Autodesk Fusion 360 part; units mm, degrees
note: some values were not read from the file. Chosen so that the rebuilt part matches the saved one: which face or edge a step refers to; which pieces of a blend or face edit are solid. Set by a fixed rule: which sketch regions a step uses.
(part 4 of 5)
  line L270 (74.1186, 72.7044) -> (69.1688, 67.7546)
  line L271 (49.0163, 92.8569) -> (45.9408, 89.7814)
  line L272 (61.3906, 64.2191) -> (67.0475, 69.8759)
  line L273 (69.8759, 67.0475) -> (64.2191, 61.3906)
  line L274 (70.9366, 70.9366) -> (49.0163, 92.8569)
  line L275 (56.4409, 62.0978) -> (59.9764, 65.6333)
  line L276 (70.9366, 70.9366) -> (49.0163, 92.8569)
  line L277 (69.8759, 67.0475) -> (64.2191, 61.3906)
  arc A224 (33.8135, 84.7252) -> (33.8135, 77.6541) centre (37.349, 81.1896) ccw
  arc A225 (37.0951, 88.0068) -> (35.2806, 96.2368) centre (33.5596, 91.5424) ccw
  line L278 (38.7632, 55.7338) -> (34.8741, 51.8447)
  arc A226 (37.0951, 88.0068) -> (35.2806, 96.2368) centre (33.5596, 91.5424) ccw
  arc A227 (40.8846, 84.7252) -> (40.8846, 77.6541) centre (44.4201, 81.1896) ccw
  arc A228 (40.8846, 84.7252) -> (40.8846, 77.6541) centre (44.4201, 81.1896) ccw
  line L279 (38.7632, 55.7338) -> (34.8741, 51.8447)
  line L280 (33.8135, 84.7252) -> (37.0951, 88.0068)
  line L281 (49.7234, 68.8153) -> (40.8846, 77.6541)
  line L282 (33.8135, 84.7252) -> (37.0951, 88.0068)
  arc A229 (33.8135, 84.7252) -> (33.8135, 77.6541) centre (37.349, 81.1896) ccw
  arc A230 (77.6541, 40.8846) -> (84.7252, 40.8846) centre (81.1896, 44.4201) ccw
  line L283 (49.0163, 92.8569) -> (45.9408, 89.7814)
  arc A231 (99.7259, 40.1371) -> (86.6476, 42.807) centre (92.3045, 37.1501) ccw
  line L284 (67.0475, 69.8759) -> (69.8759, 67.0475)
  arc A232 (24.049, -81.3368) -> (30.5907, -80.8769) centre (27.0551, -77.3414) ccw
  arc A233 (77.6541, 40.8846) -> (84.7252, 40.8846) centre (81.1896, 44.4201) ccw
  line L285 (88.4889, 37.5772) -> (86.1394, 35.2277)
  arc A234 (96.2368, 35.2806) -> (88.0068, 37.0951) centre (91.5424, 33.5596) ccw
  line L286 (61.3906, 64.2191) -> (67.0475, 69.8759)
  line L287 (74.1186, 72.7044) -> (69.1688, 67.7546)
  arc A235 (45.9408, 89.7814) -> (44.4738, 97.869) centre (42.4052, 93.3169) ccw
  line L288 (72.7044, 74.1186) -> (74.1186, 72.7044)
  circle A236 centre (64.2191, 64.2191) radius 1
  line L289 (92.8569, 49.0163) -> (70.9366, 70.9366)
  line L290 (49.7234, 68.8153) -> (68.8153, 49.7234)
  line L291 (65.6333, 59.9764) -> (62.0978, 56.4409)
  circle A237 centre (27.9799, -51.6679) radius 1.75
  line L292 (-80.8769, 30.5907) -> (-81.1896, 30.278)
  line L293 (-51.8447, -34.8741) -> (-34.8741, -51.8447)
  line L294 (-86.1394, 35.2277) -> (-84.7252, 33.8135)
  line L295 (-56.4409, -62.0978) -> (-40.8846, -77.6541)
  line L296 (-37.7026, -56.7945) -> (-56.7945, -37.7026)
  line L297 (-37.7026, -56.7945) -> (-56.7945, -37.7026)
  line L298 (-39.8239, -11.5396) -> (-57.5016, -29.2173)
  line L299 (-11.5396, -39.8239) -> (-39.8239, -11.5396)
  line L300 (-68.8153, -49.7234) -> (-49.7234, -68.8153)
  line L301 (-39.8239, -11.5396) -> (-57.5016, -29.2173)
  line L302 (-80.8769, 30.5907) -> (-81.1896, 30.278)
  line L303 (-30.5907, -80.8769) -> (-77.6541, -33.8135)
  arc A238 (-30.5907, -80.8769) -> (-24.049, -81.3368) centre (-27.0551, -77.3414) ccw
  line L304 (-29.2173, -57.5016) -> (-11.5396, -39.8239)
  line L305 (-11.5396, -39.8239) -> (-39.8239, -11.5396)
  line L306 (-57.5016, -29.2173) -> (-29.2173, -57.5016)
  arc A239 (-44.4738, -97.869) -> (-37.8014, -100.6345) centre (0, 0) ccw
  line L307 (-56.4409, -62.0978) -> (-40.8846, -77.6541)
  line L308 (-56.4409, -62.0978) -> (-62.0978, -56.4409)
  arc A240 (-44.4738, -97.869) -> (-37.8014, -100.6345) centre (0, 0) ccw
  line L309 (-51.8447, -34.8741) -> (-34.8741, -51.8447)
  line L310 (-49.7234, -68.8153) -> (-37.7026, -56.7945)
  line L311 (-34.8741, -51.8447) -> (-38.7632, -55.7338)
  line L312 (-30.5907, -80.8769) -> (-77.6541, -33.8135)
  line L313 (-51.8447, -34.8741) -> (-34.8741, -51.8447)
  circle A241 centre (-41.0613, -17.3733) radius 1.75
  line L314 (-34.8741, -51.8447) -> (-38.7632, -55.7338)
  line L315 (-57.5016, -29.2173) -> (-29.2173, -57.5016)
  line L316 (-38.7632, -55.7338) -> (-55.7338, -38.7632)
  line L317 (-51.8447, -34.8741) -> (-34.8741, -51.8447)
  line L318 (-38.7632, -55.7338) -> (-55.7338, -38.7632)
  line L319 (-86.1394, 35.2277) -> (-84.7252, 33.8135)
  circle A242 centre (-41.0613, -17.3733) radius 1.75
  arc A243 (-42.807, -86.6476) -> (-40.1371, -99.7259) centre (-37.1501, -92.3045) ccw
  line L320 (-29.2173, -57.5016) -> (-11.5396, -39.8239)
  line L321 (-29.2173, -57.5016) -> (-11.5396, -39.8239)
  line L322 (-34.8741, -51.8447) -> (-38.7632, -55.7338)
  circle A244 centre (-41.0613, -17.3733) radius 1.75
  line L323 (-37.7026, -56.7945) -> (-56.7945, -37.7026)
  circle A245 centre (-17.3733, -41.0613) radius 1.75
  circle A246 centre (-41.0613, -17.3733) radius 1.75
  line L324 (-11.5396, -39.8239) -> (-39.8239, -11.5396)
  line L325 (-39.8239, -11.5396) -> (-57.5016, -29.2173)
  line L326 (-51.8447, -34.8741) -> (-34.8741, -51.8447)
  line L327 (-34.8741, -51.8447) -> (-38.7632, -55.7338)
  arc A247 (-44.4738, -97.869) -> (-37.8014, -100.6345) centre (0, 0) ccw
  line L328 (-38.7632, -55.7338) -> (-55.7338, -38.7632)
  line L329 (-34.8741, -51.8447) -> (-38.7632, -55.7338)
  line L330 (-11.5396, -39.8239) -> (-39.8239, -11.5396)
  circle A248 centre (-27.9799, -51.6679) radius 1.75
  line L331 (-56.4409, -62.0978) -> (-40.8846, -77.6541)
  line L332 (-88.4889, 37.5772) -> (-86.1394, 35.2277)
  line L333 (-86.1394, 35.2277) -> (-84.7252, 33.8135)
  line L334 (-39.8239, -11.5396) -> (-57.5016, -29.2173)
  line L335 (-38.7632, -55.7338) -> (-55.7338, -38.7632)
  line L336 (-34.8741, -51.8447) -> (-38.7632, -55.7338)
  line L337 (-41.5917, -85.4323) -> (-49.0163, -92.8569)
  line L338 (-83.0899, 32.1782) -> (-81.1896, 30.278)
  line L339 (-38.7632, -55.7338) -> (-55.7338, -38.7632)
  line L340 (-34.8741, -51.8447) -> (-38.7632, -55.7338)
  line L341 (-57.5016, -29.2173) -> (-29.2173, -57.5016)
  circle A249 centre (-27.9799, -51.6679) radius 1.75
  line L342 (-38.7632, -55.7338) -> (-55.7338, -38.7632)
  circle A250 centre (-41.0613, -17.3733) radius 1.75
  arc A251 (0, -78.3) -> (-31.5378, -98.1221) centre (0, -113.3) ccw
  line L343 (-68.8153, -49.7234) -> (-49.7234, -68.8153)
  line L344 (-70.9366, -70.9366) -> (-92.8569, -49.0163)
  line L345 (-65.6333, -59.9764) -> (-59.9764, -65.6333)
  line L346 (-37.5772, -88.4889) -> (-35.2277, -86.1394)
  arc A252 (0, -78.3) -> (-31.5378, -98.1221) centre (0, -113.3) ccw
  arc A253 (-31.8637, -89.1193) -> (-35.2447, -94.3842) centre (0, -113.3) ccw
  arc A254 (0, -73.3) -> (-24.049, -81.3368) centre (0, -113.3) ccw
  circle A255 centre (-17.3733, -41.0613) radius 1.75
  arc A256 (24.049, -81.3368) -> (0, -73.3) centre (0, -113.3) ccw
  line L347 (-56.4409, -62.0978) -> (-62.0978, -56.4409)
  line L348 (-68.8153, -49.7234) -> (-49.7234, -68.8153)
  line L349 (-56.4409, -62.0978) -> (-62.0978, -56.4409)
  arc A257 (0, -73.3) -> (-24.049, -81.3368) centre (0, -113.3) ccw
  line L350 (-41.5917, -85.4323) -> (-40.8846, -84.7252)
  line L351 (-32.3993, -86.1394) -> (-32.0426, -86.496)
  arc A258 (-31.8637, -89.1193) -> (-35.2447, -94.3842) centre (0, -113.3) ccw
  line L352 (-65.6333, -59.9764) -> (-59.9764, -65.6333)
  line L353 (-56.4409, -62.0978) -> (-62.0978, -56.4409)
  circle A259 centre (-17.3733, -41.0613) radius 1.75
  arc A260 (-31.8637, -89.1193) -> (-35.2447, -94.3842) centre (0, -113.3) ccw
  arc A261 (24.049, -81.3368) -> (0, -73.3) centre (0, -113.3) ccw
  arc A262 (0, -73.3) -> (-24.049, -81.3368) centre (0, -113.3) ccw
  line L354 (-37.5772, -88.4889) -> (-40.3326, -91.2443)
  line L355 (-68.8153, -49.7234) -> (-49.7234, -68.8153)
  line L356 (-65.6333, -59.9764) -> (-59.9764, -65.6333)
  line L357 (-56.4409, -62.0978) -> (-62.0978, -56.4409)
  line L358 (-65.6333, -59.9764) -> (-59.9764, -65.6333)
  line L359 (-70.9366, -70.9366) -> (-92.8569, -49.0163)
  line L360 (-70.9366, -70.9366) -> (-92.8569, -49.0163)
  arc A263 (24.049, -81.3368) -> (0, -73.3) centre (0, -113.3) ccw
  arc A264 (24.049, -81.3368) -> (0, -73.3) centre (0, -113.3) ccw
  circle A265 centre (-27.9799, -51.6679) radius 1.75
  arc A266 (-31.321, -97.5974) -> (-31.2855, -97.6087) centre (0, 0) ccw
  line L361 (-29.2173, -57.5016) -> (-11.5396, -39.8239)
  line L362 (-65.6333, -59.9764) -> (-59.9764, -65.6333)
  circle A267 centre (-17.3733, -41.0613) radius 1.75
  circle A268 centre (-27.9799, -51.6679) radius 1.75
  line L363 (-37.5772, -88.4889) -> (-40.3326, -91.2443)
  line L364 (-68.8153, -49.7234) -> (-49.7234, -68.8153)
  arc A269 (0, -73.3) -> (-24.049, -81.3368) centre (0, -113.3) ccw
  line L365 (-70.9366, -70.9366) -> (-92.8569, -49.0163)
  line L366 (-37.5772, -88.4889) -> (-40.3326, -91.2443)
  arc A270 (0, -73.3) -> (-24.049, -81.3368) centre (0, -113.3) ccw
  line L367 (-37.5772, -88.4889) -> (-40.3326, -91.2443)
  arc A271 (-30.5907, -80.8769) -> (-24.049, -81.3368) centre (-27.0551, -77.3414) ccw
  line L368 (-65.6333, -59.9764) -> (-59.9764, -65.6333)
  arc A272 (0, -73.3) -> (-24.049, -81.3368) centre (0, -113.3) ccw
  arc A273 (-40.8846, -84.7252) -> (-40.8846, -77.6541) centre (-44.4201, -81.1896) ccw
  line L369 (-68.8153, -49.7234) -> (-49.7234, -68.8153)
  line L370 (-65.6333, -59.9764) -> (-59.9764, -65.6333)
  line L371 (-41.5917, -85.4323) -> (-40.8846, -84.7252)
  line L372 (-34.8741, -51.8447) -> (-38.7632, -55.7338)
  arc A274 (-32.3993, -86.1394) -> (-35.2277, -86.1394) centre (-33.8135, -87.5536) ccw
  arc A275 (24.049, -81.3368) -> (0, -73.3) centre (0, -113.3) ccw
  arc A276 (-31.8637, -89.1193) -> (-35.2447, -94.3842) centre (0, -113.3) ccw
  arc A277 (24.049, -81.3368) -> (0, -73.3) centre (0, -113.3) ccw
  arc A278 (-37.7434, -95.2979) -> (-35.2447, -94.3842) centre (-37.007, -93.4384) ccw
  arc A279 (-37.9256, -100.5859) -> (-37.9262, -100.5876) centre (0, -113.3) ccw
  line L373 (-65.6333, -59.9764) -> (-59.9764, -65.6333)
  line L374 (-68.8153, -49.7234) -> (-49.7234, -68.8153)
  line L375 (-56.4409, -62.0978) -> (-62.0978, -56.4409)
  line L376 (-38.7632, -55.7338) -> (-55.7338, -38.7632)
  line L377 (-56.4409, -62.0978) -> (-62.0978, -56.4409)
  arc A280 (-40.3326, -91.2443) -> (-39.6929, -94.5025) centre (-38.9184, -92.6585) ccw
  arc A281 (-40.8846, -84.7252) -> (-40.8846, -77.6541) centre (-44.4201, -81.1896) ccw
  arc A282 (-37.9256, -100.5859) -> (-37.9262, -100.5876) centre (0, -113.3) ccw
  line L378 (-56.7945, -37.7026) -> (-68.8153, -49.7234)
  line L379 (-37.5772, -88.4889) -> (-35.2277, -86.1394)
  line L380 (-59.9764, -65.6333) -> (-56.4409, -62.0978)
  arc A283 (-40.3326, -91.2443) -> (-39.6929, -94.5025) centre (-38.9184, -92.6585) ccw
  arc A284 (-31.8637, -89.1193) -> (-32.0426, -86.496) centre (-33.4568, -87.9102) ccw
  arc A285 (-31.8637, -89.1193) -> (-32.0426, -86.496) centre (-33.4568, -87.9102) ccw
  arc A286 (-37.9256, -100.5859) -> (-37.9262, -100.5876) centre (0, -113.3) ccw
  arc A287 (-37.9256, -100.5859) -> (-37.9262, -100.5876) centre (0, -113.3) ccw
  line L381 (-56.7945, -37.7026) -> (-68.8153, -49.7234)
  arc A288 (-39.6929, -94.5025) -> (-37.7434, -95.2979) centre (0, 0) ccw
  arc A289 (-39.6929, -94.5025) -> (-37.7434, -95.2979) centre (0, 0) ccw
  line L382 (-59.9764, -65.6333) -> (-56.4409, -62.0978)
  arc A290 (-32.3993, -86.1394) -> (-35.2277, -86.1394) centre (-33.8135, -87.5536) ccw
  line L383 (-69.8759, -67.0475) -> (-67.0475, -69.8759)
  line L384 (-56.7945, -37.7026) -> (-68.8153, -49.7234)
  arc A291 (-37.7434, -95.2979) -> (-35.2447, -94.3842) centre (-37.007, -93.4384) ccw
  line L385 (-56.7945, -37.7026) -> (-68.8153, -49.7234)
  arc A292 (-32.3993, -86.1394) -> (-35.2277, -86.1394) centre (-33.8135, -87.5536) ccw
  line L386 (-56.7945, -37.7026) -> (-68.8153, -49.7234)
  line L387 (-56.7945, -37.7026) -> (-68.8153, -49.7234)
  line L388 (-59.9764, -65.6333) -> (-56.4409, -62.0978)
  line L389 (-49.0163, -92.8569) -> (-70.9366, -70.9366)
  line L390 (-68.8153, -49.7234) -> (-49.7234, -68.8153)
  line L391 (-59.9764, -65.6333) -> (-56.4409, -62.0978)
  line L392 (-49.0163, -92.8569) -> (-45.9408, -89.7814)
  arc A293 (-31.8637, -89.1193) -> (-32.0426, -86.496) centre (-33.4568, -87.9102) ccw
  line L393 (-41.5917, -85.4323) -> (-40.8846, -84.7252)
  line L394 (-59.9764, -65.6333) -> (-56.4409, -62.0978)
  line L395 (-49.0163, -92.8569) -> (-70.9366, -70.9366)
  arc A294 (-39.6929, -94.5025) -> (-37.7434, -95.2979) centre (0, 0) ccw
  line L396 (-56.7945, -37.7026) -> (-68.8153, -49.7234)
  line L397 (-64.2191, -61.3906) -> (-69.8759, -67.0475)
  line L398 (-59.9764, -65.6333) -> (-56.4409, -62.0978)
  arc A295 (-37.9256, -100.5859) -> (-37.9262, -100.5876) centre (0, -113.3) ccw
  arc A296 (-40.3326, -91.2443) -> (-39.6929, -94.5025) centre (-38.9184, -92.6585) ccw
  line L399 (-32.3993, -86.1394) -> (-32.0426, -86.496)
  line L400 (-49.0163, -92.8569) -> (-70.9366, -70.9366)
  arc A297 (-37.7434, -95.2979) -> (-35.2447, -94.3842) centre (-37.007, -93.4384) ccw
  line L401 (-41.5917, -85.4323) -> (-40.8846, -84.7252)
  arc A298 (-39.6929, -94.5025) -> (-37.7434, -95.2979) centre (0, 0) ccw
  arc A299 (-37.9256, -100.5859) -> (-37.9262, -100.5876) centre (0, -113.3) ccw
  line L402 (-59.9764, -65.6333) -> (-56.4409, -62.0978)
  line L403 (-37.5772, -88.4889) -> (-35.2277, -86.1394)
  arc A300 (-37.7434, -95.2979) -> (-35.2447, -94.3842) centre (-37.007, -93.4384) ccw
  arc A301 (-40.8846, -84.7252) -> (-40.8846, -77.6541) centre (-44.4201, -81.1896) ccw
  arc A302 (-40.3326, -91.2443) -> (-39.6929, -94.5025) centre (-38.9184, -92.6585) ccw
  arc A303 (-32.3993, -86.1394) -> (-35.2277, -86.1394) centre (-33.8135, -87.5536) ccw
  arc A304 (-31.8637, -89.1193) -> (-32.0426, -86.496) centre (-33.4568, -87.9102) ccw
  line L404 (-37.5772, -88.4889) -> (-35.2277, -86.1394)
  arc A305 (-31.321, -97.5974) -> (-31.2855, -97.6087) centre (0, 0) ccw
  line L405 (-56.7945, -37.7026) -> (-68.8153, -49.7234)
  line L406 (-49.0163, -92.8569) -> (-70.9366, -70.9366)
  line L407 (-32.3993, -86.1394) -> (-32.0426, -86.496)
  line L408 (-64.2191, -61.3906) -> (-69.8759, -67.0475)
  line L409 (-56.4409, -62.0978) -> (-62.0978, -56.4409)
  line L410 (-32.3993, -86.1394) -> (-32.0426, -86.496)
  arc A306 (-40.8846, -84.7252) -> (-40.8846, -77.6541) centre (-44.4201, -81.1896) ccw
  line L411 (-49.0163, -92.8569) -> (-42.807, -86.6476)
  circle A307 centre (-51.6679, -27.9799) radius 1.75
  arc A308 (-45.9408, -89.7814) -> (-44.4738, -97.869) centre (-42.4052, -93.3169) ccw
  arc A309 (-37.9256, -100.5859) -> (-37.9262, -100.5876) centre (0, -113.3) ccw
  arc A310 (-31.321, -97.5974) -> (-31.2855, -97.6087) centre (0, 0) ccw
  line L412 (-55.7338, -38.7632) -> (-51.8447, -34.8741)
  arc A311 (-37.9256, -100.5859) -> (-31.321, -97.5974) centre (-36.0432, -95.9538) ccw
  circle A312 centre (-51.6679, -27.9799) radius 1.75
  line L413 (-55.7338, -38.7632) -> (-51.8447, -34.8741)
  arc A313 (-31.321, -97.5974) -> (-31.2855, -97.6087) centre (0, 0) ccw
  line L414 (-64.2191, -61.3906) -> (-69.8759, -67.0475)
  line L415 (-92.8569, -49.0163) -> (-84.7252, -40.8846)
  line L416 (-69.8759, -67.0475) -> (-67.0475, -69.8759)
  line L417 (-92.8569, -49.0163) -> (-84.7252, -40.8846)
  line L418 (-64.2191, -61.3906) -> (-69.8759, -67.0475)
  line L419 (-92.8569, -49.0163) -> (-84.7252, -40.8846)
  arc A314 (-31.321, -97.5974) -> (-31.2855, -97.6087) centre (0, 0) ccw
  line L420 (-49.0163, -92.8569) -> (-45.9408, -89.7814)
  arc A315 (-96.2368, -35.2806) -> (-88.0068, -37.0951) centre (-91.5424, -33.5596) ccw
  line L421 (-69.8759, -67.0475) -> (-67.0475, -69.8759)
  arc A316 (-37.9256, -100.5859) -> (-37.9262, -100.5876) centre (0, -113.3) ccw
  line L422 (-55.7338, -38.7632) -> (-51.8447, -34.8741)
  line L423 (-92.8569, -49.0163) -> (-86.6476, -42.807)
  line L424 (-64.2191, -61.3906) -> (-69.8759, -67.0475)
  line L425 (-49.0163, -92.8569) -> (-45.9408, -89.7814)
  arc A317 (-45.9408, -89.7814) -> (-44.4738, -97.869) centre (-42.4052, -93.3169) ccw
  line L426 (-84.7252, -33.8135) -> (-88.0068, -37.0951)
  line L427 (-55.7338, -38.7632) -> (-51.8447, -34.8741)
  line L428 (-55.7338, -38.7632) -> (-51.8447, -34.8741)
  circle A318 centre (-64.2191, -64.2191) radius 1
  line L429 (-55.7338, -38.7632) -> (-51.8447, -34.8741)
  line L430 (-67.0475, -69.8759) -> (-61.3906, -64.2191)
  arc A319 (-37.9256, -100.5859) -> (-37.9262, -100.5876) centre (0, -113.3) ccw
  line L431 (-69.8759, -67.0475) -> (-67.0475, -69.8759)
  circle A320 centre (-51.6679, -27.9799) radius 1.75
  line L432 (-49.0163, -92.8569) -> (-45.9408, -89.7814)
  circle A321 centre (-51.6679, -27.9799) radius 1.75
  line L433 (-84.7252, -33.8135) -> (-88.0068, -37.0951)
  arc A322 (-31.321, -97.5974) -> (-31.2855, -97.6087) centre (0, 0) ccw
  arc A323 (-37.9256, -100.5859) -> (-31.321, -97.5974) centre (-36.0432, -95.9538) ccw
  arc A324 (-45.9408, -89.7814) -> (-44.4738, -97.869) centre (-42.4052, -93.3169) ccw
  line L434 (-92.8569, -49.0163) -> (-85.4323, -41.5917)
  circle A325 centre (-51.6679, -27.9799) radius 1.75
  line L435 (-69.8759, -67.0475) -> (-67.0475, -69.8759)
  arc A326 (-37.9256, -100.5859) -> (-37.9262, -100.5876) centre (0, -113.3) ccw
  line L436 (-69.8759, -67.0475) -> (-67.0475, -69.8759)
  line L437 (-59.9764, -65.6333) -> (-56.4409, -62.0978)
  line L438 (-84.7252, -33.8135) -> (-88.0068, -37.0951)
  line L439 (-69.8759, -67.0475) -> (-67.0475, -69.8759)
  line L440 (-55.7338, -38.7632) -> (-51.8447, -34.8741)
  line L441 (-69.8759, -67.0475) -> (-67.0475, -69.8759)
  line L442 (-64.2191, -61.3906) -> (-69.8759, -67.0475)
  arc A327 (-37.9256, -100.5859) -> (-37.9262, -100.5876) centre (0, -113.3) ccw
  circle A328 centre (-51.6679, -27.9799) radius 1.75
  circle A329 centre (-51.6679, -27.9799) radius 1.75
  arc A330 (-31.321, -97.5974) -> (-31.2855, -97.6087) centre (0, 0) ccw
  arc A331 (-37.9256, -100.5859) -> (-37.9262, -100.5876) centre (0, -113.3) ccw
  line L443 (-92.8569, -49.0163) -> (-85.4323, -41.5917)
  arc A332 (-45.9408, -89.7814) -> (-44.4738, -97.869) centre (-42.4052, -93.3169) ccw
  arc A333 (-37.9256, -100.5859) -> (-31.321, -97.5974) centre (-36.0432, -95.9538) ccw
  arc A334 (-31.321, -97.5974) -> (-31.2855, -97.6087) centre (0, 0) ccw
  line L444 (-92.8569, -49.0163) -> (-85.4323, -41.5917)
  arc A335 (-37.9256, -100.5859) -> (-31.321, -97.5974) centre (-36.0432, -95.9538) ccw
  arc A336 (-96.2368, -35.2806) -> (-88.0068, -37.0951) centre (-91.5424, -33.5596) ccw
  line L445 (-64.2191, -61.3906) -> (-69.8759, -67.0475)
  line L446 (-55.7338, -38.7632) -> (-51.8447, -34.8741)
  circle A337 centre (-51.6679, -27.9799) radius 1.75
  line L447 (-64.2191, -61.3906) -> (-69.8759, -67.0475)
  circle A338 centre (-64.2191, -64.2191) radius 1
  line L448 (-61.3906, -64.2191) -> (-64.2191, -61.3906)
  arc A339 (-96.2368, -35.2806) -> (-88.0068, -37.0951) centre (-91.5424, -33.5596) ccw
  line L449 (-61.3906, -64.2191) -> (-64.2191, -61.3906)
  circle A340 centre (-64.2191, -64.2191) radius 1
  line L450 (-92.8569, -49.0163) -> (-89.7814, -45.9408)
  line L451 (-61.3906, -64.2191) -> (-64.2191, -61.3906)
  line L452 (-69.1688, -67.7546) -> (-74.1186, -72.7044)
  arc A341 (-97.869, -44.4738) -> (-89.7814, -45.9408) centre (-93.3169, -42.4052) ccw
  line L453 (-61.3906, -64.2191) -> (-64.2191, -61.3906)
  line L454 (-62.0978, -56.4409) -> (-65.6333, -59.9764)
  line L455 (-69.1688, -67.7546) -> (-74.1186, -72.7044)
  line L456 (-67.0475, -69.8759) -> (-61.3906, -64.2191)
  line L457 (-62.0978, -56.4409) -> (-65.6333, -59.9764)
  line L458 (-72.7044, -74.1186) -> (-67.7546, -69.1688)
  line L459 (-62.0978, -56.4409) -> (-65.6333, -59.9764)
  circle A342 centre (-64.2191, -64.2191) radius 1
  line L460 (-72.7044, -74.1186) -> (-67.7546, -69.1688)
  line L461 (-69.1688, -67.7546) -> (-74.1186, -72.7044)
  line L462 (-67.0475, -69.8759) -> (-61.3906, -64.2191)
  line L463 (-62.0978, -56.4409) -> (-65.6333, -59.9764)
  line L464 (-72.7044, -74.1186) -> (-67.7546, -69.1688)
  line L465 (-68.8153, -49.7234) -> (-77.6541, -40.8846)
  line L466 (-62.0978, -56.4409) -> (-65.6333, -59.9764)
  arc A343 (-96.2368, -35.2806) -> (-88.0068, -37.0951) centre (-91.5424, -33.5596) ccw
  arc A344 (-97.869, -44.4738) -> (-89.7814, -45.9408) centre (-93.3169, -42.4052) ccw
  line L467 (-70.2295, -71.6437) -> (-71.6437, -70.2295)
  line L468 (-70.2295, -71.6437) -> (-71.6437, -70.2295)
  arc A345 (-97.869, -44.4738) -> (-89.7814, -45.9408) centre (-93.3169, -42.4052) ccw
  line L469 (-61.3906, -64.2191) -> (-64.2191, -61.3906)
  line L470 (-92.8569, -49.0163) -> (-84.7252, -40.8846)
  arc A346 (-99.7259, -40.1371) -> (-86.6476, -42.807) centre (-92.3045, -37.1501) ccw
  line L471 (-62.0978, -56.4409) -> (-65.6333, -59.9764)
  line L472 (-70.2295, -71.6437) -> (-71.6437, -70.2295)
  circle A347 centre (-64.2191, -64.2191) radius 1
  line L473 (-69.1688, -67.7546) -> (-74.1186, -72.7044)
  line L474 (-67.0475, -69.8759) -> (-61.3906, -64.2191)
  circle A348 centre (-64.2191, -64.2191) radius 1
  line L475 (-61.3906, -64.2191) -> (-64.2191, -61.3906)
  circle A349 centre (-64.2191, -64.2191) radius 1
  line L476 (-72.7044, -74.1186) -> (-67.7546, -69.1688)
  line L477 (-68.8153, -49.7234) -> (-77.6541, -40.8846)
  line L478 (-61.3906, -64.2191) -> (-64.2191, -61.3906)
  arc A350 (-77.6541, -40.8846) -> (-84.7252, -40.8846) centre (-81.1896, -44.4201) ccw
  line L479 (-72.7044, -74.1186) -> (-67.7546, -69.1688)
  line L480 (-67.0475, -69.8759) -> (-61.3906, -64.2191)
  line L481 (-62.0978, -56.4409) -> (-65.6333, -59.9764)
  line L482 (-69.1688, -67.7546) -> (-74.1186, -72.7044)
  line L483 (-84.7252, -33.8135) -> (-88.0068, -37.0951)
  line L484 (-67.0475, -69.8759) -> (-61.3906, -64.2191)
  arc A351 (-77.6541, -33.8135) -> (-84.7252, -33.8135) centre (-81.1896, -37.349) ccw
  line L485 (-61.3906, -64.2191) -> (-64.2191, -61.3906)
  line L486 (-62.0978, -56.4409) -> (-65.6333, -59.9764)
  line L487 (-70.2295, -71.6437) -> (-71.6437, -70.2295)
  line L488 (-92.8569, -49.0163) -> (-89.7814, -45.9408)
  line L489 (-69.1688, -67.7546) -> (-74.1186, -72.7044)
  arc A352 (-77.6541, -33.8135) -> (-84.7252, -33.8135) centre (-81.1896, -37.349) ccw
  line L490 (-69.1688, -67.7546) -> (-74.1186, -72.7044)
  arc A353 (-77.6541, -40.8846) -> (-84.7252, -40.8846) centre (-81.1896, -44.4201) ccw
  line L491 (-67.0475, -69.8759) -> (-61.3906, -64.2191)
  line L492 (-69.1688, -67.7546) -> (-74.1186, -72.7044)
  line L493 (-72.7044, -74.1186) -> (-67.7546, -69.1688)
  circle A354 centre (-64.2191, -64.2191) radius 1
  line L494 (-68.8153, -49.7234) -> (-77.6541, -40.8846)
  line L495 (-68.8153, -49.7234) -> (-77.6541, -40.8846)
  arc A355 (-97.869, -44.4738) -> (-89.7814, -45.9408) centre (-93.3169, -42.4052) ccw
  line L496 (-67.7546, -69.1688) -> (-69.1688, -67.7546)
  line L497 (-72.7044, -74.1186) -> (-70.2295, -71.6437)
  line L498 (-67.7546, -69.1688) -> (-69.1688, -67.7546)
  line L499 (-74.1186, -72.7044) -> (-72.7044, -74.1186)
  line L500 (-67.0475, -69.8759) -> (-61.3906, -64.2191)
  line L501 (-72.7044, -74.1186) -> (-67.7546, -69.1688)
  arc A356 (-77.6541, -40.8846) -> (-84.7252, -40.8846) centre (-81.1896, -44.4201) ccw
  arc A357 (-77.6541, -33.8135) -> (-84.7252, -33.8135) centre (-81.1896, -37.349) ccw
  line L502 (-72.7044, -74.1186) -> (-70.2295, -71.6437)
  line L503 (-92.8569, -49.0163) -> (-85.4323, -41.5917)
  line L504 (-74.1186, -72.7044) -> (-72.7044, -74.1186)
  line L505 (-74.1186, -72.7044) -> (-72.7044, -74.1186)
  line L506 (-67.7546, -69.1688) -> (-69.1688, -67.7546)
  arc A358 (-77.6541, -33.8135) -> (-84.7252, -33.8135) centre (-81.1896, -37.349) ccw
  line L507 (-67.7546, -69.1688) -> (-69.1688, -67.7546)
  line L508 (-67.7546, -69.1688) -> (-69.1688, -67.7546)
  line L509 (-67.7546, -69.1688) -> (-69.1688, -67.7546)
  line L510 (-74.1186, -72.7044) -> (-72.7044, -74.1186)
  line L511 (-72.7044, -74.1186) -> (-70.2295, -71.6437)
  line L512 (-92.8569, -49.0163) -> (-89.7814, -45.9408)
  line L513 (-74.1186, -72.7044) -> (-72.7044, -74.1186)
  arc A359 (-77.6541, -40.8846) -> (-84.7252, -40.8846) centre (-81.1896, -44.4201) ccw
  line L514 (-67.7546, -69.1688) -> (-69.1688, -67.7546)
  line L515 (-74.1186, -72.7044) -> (-72.7044, -74.1186)
  line L516 (-72.7044, -74.1186) -> (-67.7546, -69.1688)
  line L517 (-92.8569, -49.0163) -> (-89.7814, -45.9408)
  line L518 (-74.1186, -72.7044) -> (-72.7044, -74.1186)
  line L519 (-67.7546, -69.1688) -> (-69.1688, -67.7546)
  line L520 (-74.1186, -72.7044) -> (-72.7044, -74.1186)
  line L521 (-72.7044, -74.1186) -> (-70.2295, -71.6437)
  line L522 (69.8759, -67.0475) -> (67.0475, -69.8759)
  circle A360 centre (-27.9799, 51.6679) radius 1.75
  line L523 (-92.8569, 49.0163) -> (-70.9366, 70.9366)
  line L524 (69.1688, -67.7546) -> (74.1186, -72.7044)
  line L525 (-69.8759, 67.0475) -> (-64.2191, 61.3906)
  line L526 (-33.8135, 16.8429) -> (-34.167, 17.1965)
  line L527 (-61.3906, 64.2191) -> (-67.0475, 69.8759)
  line L528 (-62.0978, 56.4409) -> (-77.6541, 40.8846)
  arc A361 (-44.4738, -97.869) -> (-37.8014, -100.6345) centre (0, 0) ccw
  line L529 (-65.6333, 59.9764) -> (-62.0978, 56.4409)
  circle A362 centre (-41.0613, -17.3733) radius 1.75
  arc A363 (44.4738, -97.869) -> (45.9408, -89.7814) centre (42.4052, -93.3169) ccw
  arc A364 (-40.8846, 77.6541) -> (-40.8846, 84.7252) centre (-44.4201, 81.1896) ccw
  line L530 (62.0978, -56.4409) -> (65.6333, -59.9764)
  arc A365 (37.7434, -95.2979) -> (39.6929, -94.5025) centre (0, 0) ccw
  line L531 (-49.7234, -68.8153) -> (-37.7026, -56.7945)
  line L532 (67.0475, -69.8759) -> (61.3906, -64.2191)
  line L533 (-11.5396, 39.8239) -> (-29.2173, 57.5016)
  line L534 (-69.8759, 67.0475) -> (-64.2191, 61.3906)
  circle A366 centre (-27.9799, 51.6679) radius 1.75
  arc A367 (37.8014, -100.6345) -> (44.4738, -97.869) centre (0, 0) ccw
  line L535 (69.8759, -67.0475) -> (67.0475, -69.8759)
  arc A368 (39.6929, -94.5025) -> (40.3326, -91.2443) centre (38.9184, -92.6585) ccw
  line L536 (41.5917, -85.4323) -> (40.8846, -84.7252)
  line L537 (-92.8569, 49.0163) -> (-70.9366, 70.9366)
  line L538 (16.8429, -33.8135) -> (17.1965, -34.167)
  circle A369 centre (-51.6679, 27.9799) radius 1.75
  line L539 (-59.9764, 65.6333) -> (-65.6333, 59.9764)
  arc A370 (0, 107.5) -> (-44.4738, 97.869) centre (0, 0) ccw
  line L540 (41.5917, -85.4323) -> (49.0163, -92.8569)
  line L541 (49.0163, -92.8569) -> (45.9408, -89.7814)
  line L542 (-49.0163, 92.8569) -> (-45.9408, 89.7814)
  line L543 (-56.4409, 62.0978) -> (-59.9764, 65.6333)
  line L544 (16.8429, -33.8135) -> (17.1965, -34.167)
  circle A371 centre (-51.6679, 27.9799) radius 1.75
  line L545 (61.3906, -64.2191) -> (64.2191, -61.3906)
  line L546 (69.8759, -67.0475) -> (67.0475, -69.8759)
  line L547 (41.5917, -85.4323) -> (40.8846, -84.7252)
  line L548 (-16.8429, 33.8135) -> (-33.8135, 16.8429)
  arc A372 (44.4738, -97.869) -> (45.9408, -89.7814) centre (42.4052, -93.3169) ccw
  line L549 (67.0475, -69.8759) -> (61.3906, -64.2191)
  line L550 (61.3906, -64.2191) -> (64.2191, -61.3906)
  line L551 (-49.0163, 92.8569) -> (-42.807, 86.6476)
  line L552 (67.0475, -69.8759) -> (61.3906, -64.2191)
  line L553 (-38.7632, 55.7338) -> (-34.8741, 51.8447)
  circle A373 centre (17.3733, -41.0613) radius 1.75
  line L554 (-49.7234, 68.8153) -> (-40.8846, 77.6541)
  line L555 (69.8759, -67.0475) -> (67.0475, -69.8759)
  line L556 (-33.8135, 16.8429) -> (-34.167, 17.1965)
  line L557 (67.0475, -69.8759) -> (61.3906, -64.2191)
  arc A374 (-46.9055, 91.138) -> (-47.1639, 91.0045) centre (0, 0) ccw
  arc A375 (37.8014, -100.6345) -> (44.4738, -97.869) centre (0, 0) ccw
  line L558 (62.0978, -56.4409) -> (65.6333, -59.9764)
  line L559 (-59.9764, 65.6333) -> (-65.6333, 59.9764)
  line L560 (-49.0163, 92.8569) -> (-40.8846, 84.7252)
  circle A376 centre (17.3733, -41.0613) radius 1.75
  line L561 (-33.8135, 84.7252) -> (-37.0951, 88.0068)
  line L562 (37.5772, -88.4889) -> (40.3326, -91.2443)
  arc A377 (40.1371, -99.7259) -> (42.807, -86.6476) centre (37.1501, -92.3045) ccw
  arc A378 (-40.1371, 99.7259) -> (-42.807, 86.6476) centre (-37.1501, 92.3045) ccw
  line L563 (62.0978, -56.4409) -> (65.6333, -59.9764)
  arc A379 (39.6929, -94.5025) -> (40.3326, -91.2443) centre (38.9184, -92.6585) ccw
  line L564 (-69.8759, 67.0475) -> (-64.2191, 61.3906)
  line L565 (67.7546, -69.1688) -> (69.1688, -67.7546)
  line L566 (-51.8447, 34.8741) -> (-55.7338, 38.7632)
  circle A380 centre (-41.0613, -17.3733) radius 1.75
  line L567 (-51.8447, 34.8741) -> (-55.7338, 38.7632)
  line L568 (67.7546, -69.1688) -> (69.1688, -67.7546)
  line L569 (61.3906, -64.2191) -> (64.2191, -61.3906)
  arc A381 (0, 107.5) -> (-44.4738, 97.869) centre (0, 0) ccw
  circle A382 centre (-51.6679, 27.9799) radius 1.75
  arc A383 (-40.8846, 77.6541) -> (-40.8846, 84.7252) centre (-44.4201, 81.1896) ccw
  line L570 (64.2191, -61.3906) -> (69.8759, -67.0475)
  arc A384 (-35.2806, 96.2368) -> (-37.0951, 88.0068) centre (-33.5596, 91.5424) ccw
  line L571 (-38.7632, 55.7338) -> (-34.8741, 51.8447)
  line L572 (-33.8135, 16.8429) -> (-34.167, 17.1965)
  line L573 (-67.0475, 69.8759) -> (-69.8759, 67.0475)
  arc A385 (35.2447, -94.3842) -> (31.8637, -89.1193) centre (0, -113.3) ccw
  line L574 (64.2191, -61.3906) -> (69.8759, -67.0475)
  line L575 (67.7546, -69.1688) -> (69.1688, -67.7546)
  line L576 (-51.8447, 34.8741) -> (-55.7338, 38.7632)
  line L577 (61.3906, -64.2191) -> (64.2191, -61.3906)
  line L578 (-59.9764, 65.6333) -> (-65.6333, 59.9764)
  arc A386 (-44.4738, 97.869) -> (-45.9408, 89.7814) centre (-42.4052, 93.3169) ccw
  circle A387 centre (17.3733, -41.0613) radius 1.75
  line L579 (-38.7632, 55.7338) -> (-34.8741, 51.8447)
  line L580 (-65.6333, 59.9764) -> (-62.0978, 56.4409)
  circle A388 centre (64.2191, -64.2191) radius 1
  line L581 (37.5772, -88.4889) -> (35.2277, -86.1394)
  circle A389 centre (64.2191, -64.2191) radius 1
  arc A390 (31.2855, -97.6087) -> (31.321, -97.5974) centre (0, 0) ccw
  line L582 (70.2295, -71.6437) -> (71.6437, -70.2295)
  arc A391 (37.9262, -100.5876) -> (37.9256, -100.5859) centre (0, -113.3) ccw
  arc A392 (-35.2806, 96.2368) -> (-37.0951, 88.0068) centre (-33.5596, 91.5424) ccw
  circle A393 centre (-51.6679, 27.9799) radius 1.75
  line L583 (70.2295, -71.6437) -> (71.6437, -70.2295)
  arc A394 (-46.9055, 91.138) -> (-47.1639, 91.0045) centre (0, 0) ccw
  line L584 (16.8429, -33.8135) -> (17.1965, -34.167)
  line L585 (-49.7234, 68.8153) -> (-40.8846, 77.6541)
  arc A395 (-33.8135, 77.6541) -> (-33.8135, 84.7252) centre (-37.349, 81.1896) ccw
  line L586 (-67.7546, 69.1688) -> (-72.7044, 74.1186)
  line L587 (64.2191, -61.3906) -> (69.8759, -67.0475)
  line L588 (62.0978, -56.4409) -> (65.6333, -59.9764)
  circle A396 centre (17.3733, -41.0613) radius 1.75
  line L589 (-38.7632, 55.7338) -> (-34.8741, 51.8447)
  line L590 (16.8429, -33.8135) -> (17.1965, -34.167)
  circle A397 centre (64.2191, -64.2191) radius 1
  line L591 (-51.8447, 34.8741) -> (-55.7338, 38.7632)
  line L592 (-61.3906, 64.2191) -> (-67.0475, 69.8759)
  arc A398 (-33.8135, 77.6541) -> (-33.8135, 84.7252) centre (-37.349, 81.1896) ccw
  line L593 (-49.0163, 92.8569) -> (-45.9408, 89.7814)
  arc A399 (0, 102.5) -> (-35.2806, 96.2368) centre (0, 0) ccw
  line L594 (-65.6333, 59.9764) -> (-62.0978, 56.4409)
  circle A400 centre (-64.2191, 64.2191) radius 1
  arc A401 (-44.4738, 97.869) -> (-45.9408, 89.7814) centre (-42.4052, 93.3169) ccw
  line L595 (49.0163, -92.8569) -> (45.9408, -89.7814)
  line L596 (-11.5396, 39.8239) -> (-29.2173, 57.5016)
  line L597 (-49.0163, 92.8569) -> (-40.8846, 84.7252)
  line L598 (64.2191, -61.3906) -> (69.8759, -67.0475)
  line L599 (-56.4409, 62.0978) -> (-59.9764, 65.6333)
  line L600 (67.7546, -69.1688) -> (69.1688, -67.7546)
  circle A402 centre (64.2191, -64.2191) radius 1
  arc A403 (0, 102.5) -> (-35.2806, 96.2368) centre (0, 0) ccw
  arc A404 (37.9262, -100.5876) -> (37.9256, -100.5859) centre (0, -113.3) ccw
  line L601 (-65.6333, 59.9764) -> (-62.0978, 56.4409)
  arc A405 (37.9262, -100.5876) -> (37.9256, -100.5859) centre (0, -113.3) ccw
  line L602 (-33.8135, 16.8429) -> (-34.167, 17.1965)
  line L603 (-67.7546, 69.1688) -> (-72.7044, 74.1186)
  arc A406 (35.2447, -94.3842) -> (37.7434, -95.2979) centre (37.007, -93.4384) ccw
  arc A407 (-84.7252, 33.8135) -> (-77.6541, 33.8135) centre (-81.1896, 37.349) ccw
  line L604 (-59.9764, 65.6333) -> (-65.6333, 59.9764)
  line L605 (-67.0475, 69.8759) -> (-69.8759, 67.0475)
  circle A408 centre (-64.2191, 64.2191) radius 1
  line L606 (-34.167, -17.1965) -> (-33.8135, -16.8429)
  line L607 (-30.5907, -80.8769) -> (-77.6541, -33.8135)
  line L608 (-34.167, -17.1965) -> (-33.8135, -16.8429)
  arc A409 (32.0426, -86.496) -> (31.8637, -89.1193) centre (33.4568, -87.9102) ccw
  arc A410 (-88.0068, 37.0951) -> (-96.2368, 35.2806) centre (-91.5424, 33.5596) ccw
  line L609 (-39.8239, -11.5396) -> (-57.5016, -29.2173)
  line L610 (-34.167, -17.1965) -> (-33.8135, -16.8429)
  arc A411 (-88.0068, 37.0951) -> (-96.2368, 35.2806) centre (-91.5424, 33.5596) ccw
  line L611 (-16.8429, -33.8135) -> (-17.1965, -34.167)
  arc A412 (-84.7252, 40.8846) -> (-77.6541, 40.8846) centre (-81.1896, 44.4201) ccw
  line L612 (-16.8429, -33.8135) -> (-17.1965, -34.167)
  line L613 (-34.167, -17.1965) -> (-33.8135, -16.8429)
  line L614 (-41.5917, -85.4323) -> (-49.0163, -92.8569)
  line L615 (-17.1965, -34.167) -> (-34.167, -17.1965)
  arc A413 (-84.7252, 40.8846) -> (-77.6541, 40.8846) centre (-81.1896, 44.4201) ccw
  arc A414 (35.2277, -86.1394) -> (32.3993, -86.1394) centre (33.8135, -87.5536) ccw
  arc A415 (31.2855, -97.6087) -> (31.321, -97.5974) centre (0, 0) ccw
  arc A416 (31.321, -97.5974) -> (37.9256, -100.5859) centre (36.0432, -95.9538) ccw
  line L616 (-72.7044, 74.1186) -> (-74.1186, 72.7044)
  arc A417 (37.9262, -100.5876) -> (37.9256, -100.5859) centre (0, -113.3) ccw
  arc A418 (35.2447, -94.3842) -> (31.8637, -89.1193) centre (0, -113.3) ccw
  arc A419 (-88.0068, 37.0951) -> (-96.2368, 35.2806) centre (-91.5424, 33.5596) ccw
  circle A420 centre (-64.2191, 64.2191) radius 1
  line L617 (-16.8429, -33.8135) -> (-17.1965, -34.167)
  arc A421 (-84.7252, 33.8135) -> (-77.6541, 33.8135) centre (-81.1896, 37.349) ccw
  circle A422 centre (-64.2191, 64.2191) radius 1
  arc A423 (32.0426, -86.496) -> (31.8637, -89.1193) centre (33.4568, -87.9102) ccw
  line L618 (32.3993, -86.1394) -> (32.0426, -86.496)
  arc A424 (-84.7252, 40.8846) -> (-77.6541, 40.8846) centre (-81.1896, 44.4201) ccw
  arc A425 (-84.7252, 40.8846) -> (-77.6541, 40.8846) centre (-81.1896, 44.4201) ccw
  line L619 (-17.1965, -34.167) -> (-34.167, -17.1965)
  arc A426 (31.2855, -97.6087) -> (31.321, -97.5974) centre (0, 0) ccw
  arc A427 (31.2855, -97.6087) -> (31.321, -97.5974) centre (0, 0) ccw
  line L620 (-34.167, -17.1965) -> (-33.8135, -16.8429)
  line L621 (-74.1186, 72.7044) -> (-69.1688, 67.7546)
  line L622 (-56.4409, 62.0978) -> (-59.9764, 65.6333)
  line L623 (-69.8759, 67.0475) -> (-64.2191, 61.3906)
  line L624 (-68.8153, 49.7234) -> (-56.7945, 37.7026)
  line L625 (-68.8153, 49.7234) -> (-56.7945, 37.7026)
  line L626 (-68.8153, 49.7234) -> (-56.7945, 37.7026)
  line L627 (-74.1186, 72.7044) -> (-69.1688, 67.7546)
  line L628 (-34.167, -17.1965) -> (-33.8135, -16.8429)
  line L629 (-49.7234, -68.8153) -> (-37.7026, -56.7945)
  line L630 (-51.8447, -34.8741) -> (-34.8741, -51.8447)
  line L631 (-34.167, -17.1965) -> (-33.8135, -16.8429)
  arc A428 (-84.7252, 33.8135) -> (-77.6541, 33.8135) centre (-81.1896, 37.349) ccw
  arc A429 (-84.7252, 33.8135) -> (-77.6541, 33.8135) centre (-81.1896, 37.349) ccw
  arc A430 (37.9262, -100.5876) -> (37.9256, -100.5859) centre (0, -113.3) ccw
  arc A431 (31.321, -97.5974) -> (37.9256, -100.5859) centre (36.0432, -95.9538) ccw
  line L632 (-39.8239, -11.5396) -> (-57.5016, -29.2173)
  line L633 (32.3993, -86.1394) -> (32.0426, -86.496)
  arc A432 (35.2447, -94.3842) -> (37.7434, -95.2979) centre (37.007, -93.4384) ccw
  line L634 (-17.1965, -34.167) -> (-34.167, -17.1965)
  line L635 (-68.8153, 49.7234) -> (-56.7945, 37.7026)
  line L636 (-56.4409, 62.0978) -> (-59.9764, 65.6333)
  arc A433 (37.9262, -100.5876) -> (37.9256, -100.5859) centre (0, -113.3) ccw
  line L637 (-72.7044, 74.1186) -> (-74.1186, 72.7044)
  line L638 (37.5772, -88.4889) -> (35.2277, -86.1394)
  arc A434 (35.2277, -86.1394) -> (32.3993, -86.1394) centre (33.8135, -87.5536) ccw
  line L639 (-85.4323, 41.5917) -> (-84.7252, 40.8846)
  line L640 (-37.7026, -56.7945) -> (-56.7945, -37.7026)
  line L641 (-85.4323, 41.5917) -> (-92.8569, 49.0163)
  line L642 (-88.4889, 37.5772) -> (-86.1394, 35.2277)
  line L643 (-80.8769, 30.5907) -> (-81.1896, 30.278)
  line L644 (-85.4323, 41.5917) -> (-92.8569, 49.0163)
  line L645 (-83.0899, 32.1782) -> (-81.1896, 30.278)
  line L646 (-88.4889, 37.5772) -> (-86.1394, 35.2277)
  line L647 (-86.1394, 35.2277) -> (-84.7252, 33.8135)
  line L648 (-16.8429, -33.8135) -> (-17.1965, -34.167)
  arc A435 (-86.6476, 42.807) -> (-99.7259, 40.1371) centre (-92.3045, 37.1501) ccw
  line L649 (-80.8769, 30.5907) -> (-81.1896, 30.278)
  line L650 (-49.7234, -68.8153) -> (-37.7026, -56.7945)
  arc A436 (-89.7814, 45.9408) -> (-97.869, 44.4738) centre (-93.3169, 42.4052) ccw
  line L651 (-92.8569, 49.0163) -> (-86.6476, 42.807)
  line L652 (-33.8135, -16.8429) -> (-16.8429, -33.8135)
  line L653 (-88.4889, 37.5772) -> (-86.1394, 35.2277)
  line L654 (-83.0899, 32.1782) -> (-81.1896, 30.278)
  line L655 (-85.4323, 41.5917) -> (-92.8569, 49.0163)
  line L656 (-85.4323, 41.5917) -> (-84.7252, 40.8846)
  line L657 (-85.4323, 41.5917) -> (-84.7252, 40.8846)
  line L658 (-85.4323, 41.5917) -> (-92.8569, 49.0163)
  line L659 (-33.8135, -16.8429) -> (-16.8429, -33.8135)
  line L660 (-34.167, -17.1965) -> (-33.8135, -16.8429)
  line L661 (-33.8135, -16.8429) -> (-16.8429, -33.8135)
  arc A437 (-88.0068, 37.0951) -> (-96.2368, 35.2806) centre (-91.5424, 33.5596) ccw
  arc A438 (-89.7814, 45.9408) -> (-97.869, 44.4738) centre (-93.3169, 42.4052) ccw
  line L662 (-85.4323, 41.5917) -> (-84.7252, 40.8846)
  line L663 (-49.7234, -68.8153) -> (-37.7026, -56.7945)
  arc A439 (-89.7814, 45.9408) -> (-97.869, 44.4738) centre (-93.3169, 42.4052) ccw
  line L664 (-83.0899, 32.1782) -> (-81.1896, 30.278)
  line L665 (-33.8135, -16.8429) -> (-16.8429, -33.8135)
  line L666 (-49.7234, -68.8153) -> (-37.7026, -56.7945)
  line L667 (-17.1965, -34.167) -> (-34.167, -17.1965)
  arc A440 (-89.7814, 45.9408) -> (-97.869, 44.4738) centre (-93.3169, 42.4052) ccw
  point P0 (-37.349, 81.1896)
  point P1 (-63.8655, -63.8655)
  point P2 (81.1896, -37.349)
  point P3 (37.349, 81.1896)
  point P4 (63.8655, -63.8655)
  point P5 (63.8655, -63.8655)
  point P6 (63.8655, -63.8655)
  point P7 (63.8655, -63.8655)
  point P8 (-63.8655, -63.8655)
  point P9 (-63.8655, -63.8655)
  point P10 (-81.1896, -37.349)
  point P11 (-63.8655, -63.8655)
  point P12 (-63.8655, -63.8655)
  point P13 (-81.1896, -37.349)
  point P14 (-63.8655, -63.8655)
  point P15 (-81.1896, -37.349)
  point P16 (63.8655, -63.8655)
  point P17 (63.8655, -63.8655)
  point P18 (63.8655, -63.8655)
  point P19 (63.8655, -63.8655)
  point P20 (-63.8655, -63.8655)
  point P21 (-63.8655, -63.8655)
  point P22 (-37.349, 81.1896)
  point P23 (37.349, 81.1896)
  point P24 (-39.8239, 11.5396)
  point P25 (-68.8153, 49.7234)
  point P26 (-61.3906, 64.2191)
  point P27 (-81.1896, -37.349)
  point P28 (-33.8135, 16.8429)
  point P29 (-63.8655, -63.8655)
  point P30 (81.1896, -37.349)
  point P31 (-63.8655, -63.8655)
  point P32 (-63.8655, -63.8655)
  point P33 (-63.8655, -63.8655)
  point P34 (-39.8239, 11.5396)
  point P35 (-63.8655, -63.8655)
  point P36 (-31.5378, -98.1221)
  point P37 (-63.8655, -63.8655)
  point P38 (-68.8153, 49.7234)
  point P39 (-63.8655, -63.8655)
  point P40 (-33.8135, 16.8429)
  point P41 (-63.8655, -63.8655)
  point P42 (-61.3906, 64.2191)
  point P43 (-31.5378, -98.1221)
  dimension "d124" = 31
  dimension "d125" = 5
  dimension "d126" = 5
  dimension "d127" = 5
  dimension "d128" = 5
  dimension "d129" = 5
  dimension "d130" = 2
  dimension "d131" = 2
  dimension "d132" = 2
  dimension "d133" = 2
  dimension "d134" = 31
  dimension "d135" = 5
  dimension "d136" = 5
  dimension "d137" = 5
  dimension "d138" = 5
  dimension "d139" = 5
  dimension "d140" = 5
  dimension "d141" = 5
  dimension "d142" = 5
  dimension "d143" = 5
  dimension "d144" = 5
  dimension "d145" = 5
  dimension "d146" = 31
  dimension "d147" = 5
  dimension "d148" = 5
  dimension "d149" = 5
  dimension "d150" = 5
  dimension "d151" = 5
  dimension "d152" = 2
  dimension "d153" = 2
  dimension "d154" = 2
  dimension "d155" = 2
  dimension "d156" = 31
  dimension "d157" = 5
  dimension "d158" = 5
  dimension "d159" = 5
  dimension "d160" = 5
  dimension "d161" = 5
  dimension "d162" = 5
  dimension "d163" = 5
  dimension "d164" = 5
  dimension "d165" = 5
  dimension "d166" = 5
  dimension "d167" = 5
  dimension "d168" = 8
  dimension "d169" = 8
  dimension "d170" = 8
  dimension "d171" = 8
  dimension "d172" = 8
  dimension "d173" = 8
  dimension "d174" = 8
  dimension "d175" = 8
  constraint concentric A277 A405
  constraint coincident L195.end L144
  constraint coincident L107.start L146
  constraint coincident L532.end L83
  constraint coincident L84.end L522
  constraint coincident L189.start L218
  constraint coincident L195.end L177
  constraint coincident L107.start L171
  constraint coincident L532.end L160
  constraint coincident L84.end L535
  constraint coincident L189.start L80
  constraint midpoint L88.end L97
  constraint midpoint L582.end L113
  constraint midpoint L128.end L583
  constraint perpendicular L135 L547
  constraint perpendicular L69 L563
  constraint perpendicular L66 L69
  constraint perpendicular L74 L166
  constraint perpendicular L128 L595
  constraint concentric A185 A367
  constraint tangent A367 A372
  constraint tangent A372 L595
  constraint concentric A193 A263
  constraint concentric A263 A391
  constraint tangent A159 L74
  constraint tangent A159 A185
  constraint tangent L75 A163
  constraint tangent A163 A201
  constraint tangent A232 A263
  constraint tangent L152 A232
  constraint coincident A190.start A404
  constraint concentric A385 A404
  constraint concentric A365 A427
  constraint perpendicular L547 L633
  constraint concentric A275 A385
  constraint coincident A21.centre L124
  constraint coincident A21.centre A365
  constraint tangent A365 A368
  constraint tangent L124 A368
  constraint coincident A416.centre A385
  constraint coincident A416.centre A365
  constraint tangent A385 A406
  constraint tangent A365 A406
  constraint tangent A385 A423
  constraint tangent A423 L633
  constraint tangent L633 A434
  constraint tangent L581 A434
  constraint coincident L234.end L264
  constraint coincident L273.end L265
  constraint coincident L270.end L262
  constraint coincident L9.end L229
  constraint perpendicular L254 L259
  constraint perpendicular L242 L281
  constraint perpendicular L276 L283
  constraint tangent L283 A235
  constraint tangent A225 L280
  constraint coincident A213.end A235
  constraint concentric A168 A201
  constraint concentric A201 A213
  constraint coincident A213.start L283
  constraint perpendicular L188 L217
  constraint parallel L188 L246
  constraint perpendicular L64 L246
  constraint concentric A185 A210
  constraint coincident P30 L66
  constraint coincident P30 L69
  constraint tangent L66 A160
  constraint tangent L69 A160
  constraint tangent A155 L152
  constraint coincident L39.end A112.start
  constraint tangent A171 L547
  constraint tangent A171 L135
  constraint coincident L64.start L217
  constraint coincident L246.start L188
  constraint tangent A153 L217
  constraint tangent A153 L188
  constraint tangent L259 A233
  constraint tangent L254 A233
  constraint coincident P23 L281
  constraint coincident P23 L242
  constraint tangent A228 L281
  constraint tangent L242 A228
  constraint tangent L217 A229
  constraint coincident A224.start L280.start
  constraint concentric A264 A433
  constraint coincident L195.end L148
  constraint coincident L107.start L170
  constraint coincident L532.end L86
  constraint coincident L84.end L546
  constraint coincident L189.start L197
  constraint coincident L195.end L182
  constraint coincident L107.start L142
  constraint coincident L532.end L153
  constraint coincident L84.end L555
  constraint coincident L189.start L191
  constraint midpoint L88.end L98
  constraint midpoint L582.end L95
  constraint midpoint L128.end L582
  constraint perpendicular L107 L536
  constraint perpendicular L76 L530
  constraint perpendicular L67 L76
  constraint perpendicular L73 L183
  constraint perpendicular L164 L541
  constraint concentric A179 A375
  constraint tangent A363 A375
  constraint tangent A363 L541
  constraint concentric A166 A256
  constraint concentric A256 A430
  constraint tangent A157 L73
  constraint tangent A157 A179
  constraint tangent A156 L72
  constraint tangent A156 A199
  constraint tangent A190 A256
  constraint tangent L168 A190
  constraint coincident A190.start A417
  constraint concentric A417 A418
  constraint concentric A177 A426
  constraint perpendicular L536 L618
  constraint concentric A261 A418
  constraint coincident A21.centre L562
  constraint coincident A21.centre A177
  constraint tangent A177 A379
  constraint tangent L562 A379
  constraint coincident A416.centre A418
  constraint coincident A416.centre A177
  constraint tangent A418 A432
  constraint tangent A177 A432
  constraint tangent A409 A418
  constraint tangent A409 L618
  constraint tangent A414 L618
  constraint tangent A414 L638
  constraint coincident L234.end L290
  constraint coincident L273.end L267
  constraint coincident L270.end L284
  constraint coincident L9.end L216
  constraint perpendicular L256 L258
  constraint perpendicular L237 L244
  constraint perpendicular L271 L274
  constraint tangent A223 L271
  constraint tangent A226 L282
  constraint coincident A213.end A223
  constraint concentric A169 A199
  constraint concentric A199 A214
  constraint coincident A213.start L271
  constraint perpendicular L203 L206
  constraint parallel L206 L250
  constraint perpendicular L247 L250
  constraint concentric A179 A203
  constraint coincident P30 L67
  constraint coincident P30 L76
  constraint tangent L67 A161
  constraint tangent A161 L76
  constraint tangent A158 L168
  constraint tangent A172 L536
  constraint tangent L107 A172
  constraint coincident L64.start L203
  constraint coincident L246.start L206
  constraint tangent L203 A219
  constraint tangent L206 A219
  constraint tangent L258 A230
  constraint tangent L256 A230
  constraint coincident P23 L237
  constraint coincident P23 L244
  constraint tangent L237 A227
  constraint tangent L244 A227
  constraint tangent L203 A224
  constraint concentric A188 A206
  constraint perpendicular L159 L551
  constraint perpendicular L537 L651
  constraint concentric A188 A191
  constraint concentric A188 A205
  constraint concentric A188 A209
  constraint tangent A191 A378
  constraint tangent L551 A378
  constraint tangent A215 L243
  constraint tangent A191 A215
  constraint tangent A205 A231
  constraint tangent L253 A231
  constraint tangent A162 A205
  constraint tangent L70 A162
  constraint tangent L90 A377
  constraint tangent A209 A377
  constraint tangent A243 L411
  constraint tangent A209 A243
  constraint tangent L423 A346
  constraint tangent A188 A346
  constraint tangent A435 L651
  constraint tangent A188 A435
  measures "d124" distance of L90.start L128.end
  measures "d125" distance of P30 L39.end
  measures "d126" radius of A372
  measures "d127" radius of A159
  measures "d128" radius of A163
  measures "d129" radius of A232
  measures "d130" radius of A368
  measures "d131" radius of A406
  measures "d132" radius of A423
  measures "d133" radius of A434
  measures "d134" distance of L252.end L263.end
  measures "d135" distance of A224.start P23
  measures "d136" radius of A221
  measures "d137" radius of A235
  measures "d138" radius of A225
  measures "d139" radius of A160
  measures "d140" radius of A155
  measures "d141" radius of A171
  measures "d142" radius of A153
  measures "d143" radius of A233
  measures "d144" radius of A228
  measures "d145" radius of A229
  measures "d146" distance of L90.start L128.end
  measures "d147" distance of L39.end P30
  measures "d148" radius of A363
  measures "d149" radius of A157
  measures "d150" radius of A156
  measures "d151" radius of A190
  measures "d152" radius of A379
  measures "d153" radius of A432
  measures "d154" radius of A409
  measures "d155" radius of A414
  measures "d156" distance of L263.end L252.end
  measures "d157" distance of P23 A224.start
  measures "d158" radius of A222
  measures "d159" radius of A223
  measures "d160" radius of A226
  measures "d161" radius of A161
  measures "d162" radius of A158
  measures "d163" radius of A172
  measures "d164" radius of A219
  measures "d165" radius of A230
  measures "d166" radius of A227
  measures "d167" radius of A224
  measures "d168" radius of A378
  measures "d169" radius of A215
  measures "d170" radius of A231
  measures "d171" radius of A162
  measures "d172" radius of A377
  measures "d173" radius of A243
  measures "d174" radius of A346
  measures "d175" radius of A435